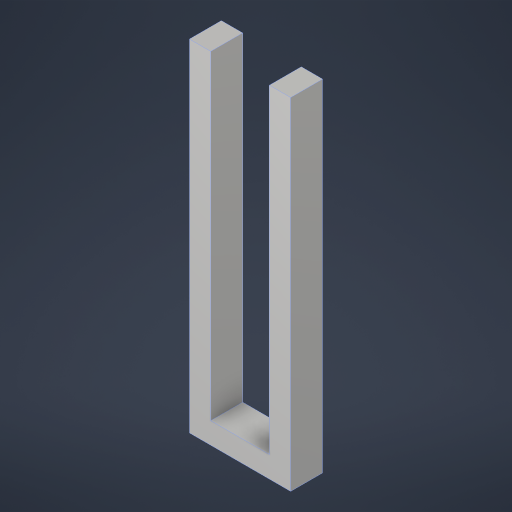
# Autodesk Inventor part: MU-006 elevator2
Saved by Autodesk Inventor 2024.2 (Build 282272000, 272)
## iProperties
Created: 2025-01-05
Part Number: MU-006 elevator2
Material: Aluminum 6061
Document SubType Name: Modeling
Designer: mavericks
Density: 2.7 g/cm^3
Appearance: Aluminum - Flat
Author: mavericks
Autodesk Inventor part; units mm, degrees
ref_plane "YZ Plane" through (0, 0, 0) normal (1, 0, 0) x (0, 1, 0)
ref_plane "XZ Plane" through (0, 0, 0) normal (0, 1, 0) x (-1, 0, 0)
ref_plane "XY Plane" through (0, 0, 0) normal (0, 0, 1) x (1, 0, 0)
sketch "Sketch1" plane through (0, 0, 0) normal (0, 0, 1) x (1, 0, 0)
  line L0 (-120.65, 812.8) -> (120.65, 812.8)
  line L1 (120.65, 812.8) -> (120.65, 0)
  line L2 (120.65, 0) -> (-120.65, 0)
  line L3 (-120.65, 0) -> (-120.65, 812.8)
  point P0 (0, 0)
  point P1 (0, 0)
  dimension "d0" = 241.3
  dimension "d1" = 812.8
  constraints: 8 end point, 2 parallel, 1 coincident, 1 horizontal, 1 midpoint, 1 perpendicular
  measures "d0" distance of L1.end L2.end
  measures "d1" distance of L2.end L0.start
extrude "Extrusion1" add sketch "Sketch1" along normal mid plane 76.2
sketch "Sketch2" plane through (0, 0, 38.1) normal (0, 0, 1) x (1, 0, 0)
  line L0 (-120.65, 0) -> (-120.65, 812.8) construction
  line L1 (-120.65, 812.8) -> (120.65, 812.8) construction
  line L2 (120.65, 812.8) -> (120.65, 0) construction
  line L3 (120.65, 0) -> (-120.65, 0) construction
  line L4 (-69.85, 812.8) -> (69.85, 812.8)
  line L5 (69.85, 812.8) -> (69.85, 50.8)
  line L6 (69.85, 50.8) -> (-69.85, 50.8)
  line L7 (-69.85, 50.8) -> (-69.85, 812.8)
  point P0 (0, 0)
  dimension "d4" = 50.8
  dimension "d5" = 50.8
  dimension "d6" = 50.8
  constraints: 8 end point, 2 parallel, 1 horizontal, 1 perpendicular, 1 point on line
  measures "d4" distance between parallel lines of L3 L6
  measures "d5" distance between parallel lines of L0 L7
  measures "d6" distance between parallel lines of L2 L5
extrude "Extrusion2" cut sketch "Sketch2" against normal through all
equation "\"d6\" = d5"
body "Solid1"
